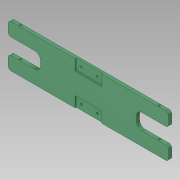
# Autodesk Inventor part: Chassis
Saved by Autodesk Inventor 2019 (Build 230136000, 136)
## iProperties
Created: 2020-03-03
Part Number: Chassis
Material: Plástico PC/ABS
Document SubType Name: Modeling
Designer: daniel.regner
Density: 0.357273 g/cm^3
Appearance: Suave - Verde mar escuro
Author: daniel.regner
Autodesk Inventor part; units mm, degrees
ref_plane "YZ Plane" through (0, 0, 0) normal (1, 0, 0) x (0, 1, 0)
ref_plane "XZ Plane" through (0, 0, 0) normal (0, 1, 0) x (-1, 0, 0)
ref_plane "XY Plane" through (0, 0, 0) normal (0, 0, 1) x (1, 0, 0)
sketch "Esboço1" plane through (0, 0, 0) normal (0, 0, 1) x (1, 0, 0)
  line L0 (145, -40) -> (-145, -40)
  line L1 (-145, 40) -> (145, 40)
  line L2 (150, -40) -> (-150, 40) construction
  line L3 (-150, -40) -> (150, 40) construction
  line L4 (-145, -15) -> (-100, -15)
  line L5 (-90, -5) -> (-90, 5)
  line L6 (-100, 15) -> (-145, 15)
  line L7 (145, 15) -> (100, 15)
  line L8 (90, 5) -> (90, -5)
  line L9 (100, -15) -> (145, -15)
  line L10 (150, 35) -> (150, 20)
  line L11 (150, -20) -> (150, -35)
  line L12 (-150, -35) -> (-150, -20)
  line L13 (-150, 20) -> (-150, 35)
  arc A0 (100, 15) -> (90, 5) centre (100, 5) ccw
  arc A1 (90, -5) -> (100, -15) centre (100, -5) ccw
  arc A2 (-100, -15) -> (-90, -5) centre (-100, -5) ccw
  arc A3 (-90, 5) -> (-100, 15) centre (-100, 5) ccw
  arc A4 (150, 35) -> (145, 40) centre (145, 35) ccw
  arc A5 (145, 15) -> (150, 20) centre (145, 20) ccw
  arc A6 (150, -20) -> (145, -15) centre (145, -20) ccw
  arc A7 (145, -40) -> (150, -35) centre (145, -35) ccw
  arc A8 (-145, -15) -> (-150, -20) centre (-145, -20) ccw
  arc A9 (-150, -35) -> (-145, -40) centre (-145, -35) ccw
  arc A10 (-145, 40) -> (-150, 35) centre (-145, 35) ccw
  arc A11 (-150, 20) -> (-145, 15) centre (-145, 20) ccw
  point P0 (0, 0)
  point P1 (-150, -15)
  point P2 (-150, 15)
  point P3 (150, 15)
  dimension "d5" = 300
  dimension "d6" = 80
  dimension "d11" = 10
  dimension "d12" = 5
  dimension "d46" = 30
  dimension "d47" = 30
  dimension "d49" = 150
  dimension "d50" = 150
  dimension "d51" = 60
  dimension "d52" = 60
  dimension "d54" = 15
  constraints: 28 end point, 25 tangent, 24 point on circle, 14 point on line, 12 centre point, 10 equal radius, 7 parallel, 4 perpendicular, 3 horizontal, 2 midpoint
  measures "d5" distance of L2.end L3.end
  measures "d6" distance between parallel lines of L0 L1
  measures "d11" radius of A0
  measures "d12" radius of A4
  measures "d46" distance between parallel lines of L4 L6
  measures "d47" distance between parallel lines of L9 L7
  measures "d49" distance from line of point (0, 0) L13
  measures "d50" distance from line of point (0, 0) L11
  measures "d51" distance between parallel lines of L11 L8
  measures "d52" distance between parallel lines of L5 L12
  measures "d54" distance from line of point (0, 0) L6
extrude "Extrusão1" add sketch "Esboço1" along normal blind 6
sketch "Esboço2" plane through (0, 0, 6) normal (0, 0, 1) x (1, 0, 0)
  line L0 (145, 40) -> (-145, 40) projected
  line L1 (25, -40) -> (-25, -40)
  line L2 (-25, 40) -> (25, 40)
  line L3 (25, -40) -> (-25, 40) construction
  line L4 (-25, -40) -> (25, 40) construction
  line L5 (-25, 20) -> (25, 20)
  line L6 (25, -20) -> (-25, -20)
  line L7 (-25, -40) -> (-25, -20)
  line L8 (-25, 20) -> (-25, 40)
  line L9 (25, 40) -> (25, 20)
  line L10 (25, -20) -> (25, -40)
  line L11 (-145, -40) -> (145, -40) projected
  point P0 (0, 0)
  dimension "d15" = 50
  dimension "d16" = 20
  dimension "d17" = 20
  dimension "d18" = 40
  dimension "d19" = 25
  dimension "d20" = 80
  constraints: 20 end point, 6 perpendicular, 5 parallel, 2 midpoint, 1 horizontal, 1 point on line
  measures "d15" distance of L2.start L2.end
  measures "d16" distance between parallel lines of L1 L6
  measures "d17" distance between parallel lines of L0 L5
  measures "d18" distance between parallel lines of L6 L5
  measures "d19" distance from line of point (0, 0) L8
  measures "d20" distance between parallel lines of L11 L0
extrude "Extrusão2" cut sketch "Esboço2" against normal blind 2
sketch "Esboço3" plane through (0, 0, 4) normal (0, 0, 1) x (1, 0, 0)
  line L0 (25, 20) -> (-25, 20) projected
  line L1 (145, 40) -> (25, 40) projected
  line L2 (32.6697, 0) -> (-36.0886, 0) construction
  point P0 (0, 0)
  point P1 (15, 30)
  point P2 (-15, 30)
  point P3 (15, -30)
  point P4 (-15, -30)
  dimension "d23" = 10
  dimension "d24" = 20
  dimension "d25" = 15
  dimension "d26" = 30
  dimension "d27" = 10
  constraints: 2 end point, 2 symmetric about line, 1 horizontal, 1 point on line
  measures "d23" distance from line of L0 point (15, 30)
  measures "d24" distance between parallel lines of L1 L0
  measures "d25" horizontal distance of point (0, 0) point (15, 30)
  measures "d26" distance of point (15, 30) point (-15, 30)
  measures "d27" distance from line of L0 point (-15, 30)
hole "Furo1" at (15, 30, 4) at (-15, 30, 4) at (15, -30, 4) at (-15, -30, 4) direction (0, 0, -1) diameter 4 end through all
sketch "Esboço4" plane through (-145, 40, 0) normal (0, 1, 0) x (1, 0, 0)
  line L0 (290, -6) -> (170, -6) projected
  line L1 (290, 0) -> (0, 0) projected
  line L2 (295, 0) -> (295, -6) projected
  line L3 (145, -28.4495) -> (145, 21.5505) construction
  point P0 (145, 0)
  point P1 (275, -3)
  point P2 (145, 0)
  point P3 (15, -3)
  dimension "d35" = 3
  dimension "d36" = 6
  dimension "d37" = 20
  dimension "d38" = 50
  constraints: 2 end point, 1 midpoint, 1 point on line, 1 symmetric about line, 1 vertical
  measures "d35" distance from line of L0 point (275, -3)
  measures "d36" distance between parallel lines of L0 L1
  measures "d37" distance from line of point (275, -3) L2
  measures "d38" distance of L3.start L3.end
hole "Furo2" at (130, 40, 3) at (-130, 40, 3) direction (0, -1, 0) diameter 4 end through all
equation "\"d47\" = d46"
equation "\"d49\" = 0.5 * d5"
equation "\"d50\" = d49"
equation "\"d52\" = d51"
equation "\"d54\" = 0.5 * d46"
equation "\"d18\" = -d17 + d20 - d16"
equation "\"d19\" = 0.5 * d15"
equation "\"d23\" = 0.5 * d24"
equation "\"d26\" = 2 * d25"
equation "\"d27\" = d23"
equation "\"d35\" = 0.5 * d36"
